Autodesk Inventor part; units mm, degrees
note: some values were not read from the file. Chosen so that the rebuilt part matches the saved one: direction of "Hole2".
(part 5 of 20)
  spline S27 degree 3 poles (-10071.861852, -10009.008209) (-10071.863963, -10009.012295) (-10071.868163, -10009.020425) (-10071.875194, -10009.032142) (-10071.882698, -10009.043397) (-10071.890711, -10009.054141) (-10071.899201, -10009.064358) (-10071.908156, -10009.074022) (-10071.917555, -10009.083111) (-10071.927381, -10009.091603) (-10071.937618, -10009.099474) (-10071.948247, -10009.1067) (-10071.95925, -10009.11326) (-10071.97061, -10009.119128) (-10071.982308, -10009.124286) (-10071.99433, -10009.128693) (-10072.006644, -10009.132397) (-10072.015041, -10009.134191) (-10072.019251, -10009.135091) knots 0 0 0 0 0.0658533 0.13104018 0.19559045 0.25953687 0.32291608 0.38576964 0.44814503 0.51009667 0.5716869 0.63298697 0.69407787 0.75505117 0.81600962 0.87706766 0.93835167 1 1 1 1
  spline S28 degree 3 poles (-10072.011557, -10009.107926) (-10072.008101, -10009.107314) (-10072.00122, -10009.106096) (-10071.991078, -10009.103593) (-10071.981148, -10009.100626) (-10071.971444, -10009.097167) (-10071.961973, -10009.093245) (-10071.949683, -10009.087429) (-10071.934919, -10009.079081) (-10071.91824, -10009.067495) (-10071.902707, -10009.054476) (-10071.888262, -10009.040263) (-10071.879682, -10009.029855) (-10071.875393, -10009.024653) knots 0 0 0 0 0.0644506 0.12832403 0.1917227 0.2547379 0.31744987 0.37992792 0.50437187 0.62845768 0.75238919 0.87624484 1 1 1 1
  spline S29 degree 3 poles (-10071.83509, -10008.810331) (-10071.836656, -10008.806851) (-10071.839768, -10008.799937) (-10071.84543, -10008.790125) (-10071.851743, -10008.780842) (-10071.858755, -10008.772119) (-10071.866422, -10008.763945) (-10071.874726, -10008.75632) (-10071.88364, -10008.749241) (-10071.89314, -10008.742705) (-10071.903202, -10008.736711) (-10071.913803, -10008.731254) (-10071.924919, -10008.726333) (-10071.936525, -10008.721945) (-10071.948599, -10008.718086) (-10071.961118, -10008.714764) (-10071.974052, -10008.711929) (-10071.982857, -10008.710502) (-10071.987308, -10008.70978) knots 0 0 0 0 0.05994656 0.11908522 0.17773662 0.23620436 0.29477068 0.35369309 0.41320222 0.47350071 0.53476324 0.59713734 0.66074485 0.72568383 0.79203056 0.85984183 0.92915698 1 1 1 1
  ellipse E534 centre (-10070.500516, -10008.838581) end of major axis (-10070.251393, -10008.817665) minor radius 0.13482 (-10070.407011, -10008.707729) -> (-10070.519101, -10008.704905) ccw
  ellipse E535 centre (-10070.496994, -10008.880539) end of major axis (-10070.746117, -10008.901455) minor radius 0.13482 (-10070.403489, -10008.749688) -> (-10070.515578, -10008.746863) ccw
  ellipse E536 centre (-10072.084336, -10008.798673) end of major axis (-10071.835212, -10008.777757) minor radius 0.13482 (-10071.990831, -10008.667822) -> (-10072.10292, -10008.664997) ccw
  ellipse E537 centre (-10072.080813, -10008.840632) end of major axis (-10072.329937, -10008.861548) minor radius 0.13482 (-10071.987308, -10008.70978) -> (-10072.099397, -10008.706956) ccw
  ellipse E538 centre (-10070.500714, -10008.942088) end of major axis (-10070.260175, -10009.010215) minor radius 0.20633 (-10070.539378, -10009.145021) -> (-10070.427738, -10009.147833) ccw
  ellipse E539 centre (-10072.084533, -10008.902181) end of major axis (-10071.843995, -10008.970307) minor radius 0.20633 (-10072.123197, -10009.105113) -> (-10072.011557, -10009.107926) ccw
  ellipse E540 centre (-10070.189892, -10008.99624) end of major axis (-10070.182637, -10008.708332) minor radius 0.048213 (-10070.237615, -10008.979123) -> (-10070.234208, -10009.15271) ccw
  ellipse E541 centre (-10070.189892, -10008.99624) end of major axis (-10070.182637, -10008.708332) minor radius 0.048213 (-10070.210183, -10008.754558) -> (-10070.231383, -10008.882208) ccw
  ellipse E542 centre (-10070.189892, -10008.99624) end of major axis (-10070.198405, -10009.334133) minor radius 0.056583 (-10070.213706, -10008.7126) -> (-10070.243358, -10008.923084) ccw
  ellipse E543 centre (-10070.189892, -10008.99624) end of major axis (-10070.198405, -10009.334133) minor radius 0.056583 (-10070.247084, -10009.05145) -> (-10070.241901, -10009.179875) ccw
  ellipse E544 centre (-10072.272412, -10008.943767) end of major axis (-10072.280926, -10009.28166) minor radius 0.056583 (-10072.296226, -10008.660127) -> (-10072.328408, -10008.92331) ccw
  ellipse E545 centre (-10072.272412, -10008.943767) end of major axis (-10072.280926, -10009.28166) minor radius 0.056583 (-10072.328363, -10009.061132) -> (-10072.324422, -10009.127402) ccw
  line L650 (-10070.153656, -10008.500579) -> (-10070.213706, -10008.7126)
  line L651 (-10072.296226, -10008.660127) -> (-10072.287518, -10008.62938)
  line L652 (-10072.262582, -10008.541339) -> (-10072.234911, -10008.443639)
  line L653 (-10070.156321, -10008.564386) -> (-10070.210183, -10008.754558)
  line L654 (-10070.55463, -10029.843391) -> (-10070.696895, -10029.517678)
  line L655 (-10070.813455, -10029.48076) -> (-10072.002453, -10029.540872)
  line L656 (-10072.082423, -10029.587726) -> (-10071.918753, -10029.962444)
  ellipse E546 centre (-10072.164414, -10029.974864) end of major axis (-10071.914557, -10029.983317) minor radius 0.10517 (-10072.058984, -10030.073195) -> (-10071.918753, -10029.962444) ccw
  line L657 (-10072.00092, -10029.495538) -> (-10070.811921, -10029.435426)
  line L658 (-10070.695362, -10029.472344) -> (-10070.552849, -10029.798623)
  line L659 (-10072.218164, -10030.077205) -> (-10072.218062, -10030.074202)
  ellipse E547 centre (-10070.79516, -10029.522646) end of major axis (-10070.695217, -10029.526028) minor radius 0.042068 (-10070.696895, -10029.517678) -> (-10070.813455, -10029.48076) ccw
  ellipse E548 centre (-10071.984158, -10029.582758) end of major axis (-10072.084101, -10029.579377) minor radius 0.042068 (-10072.002453, -10029.540872) -> (-10072.082423, -10029.587726) ccw
  ellipse E549 centre (-10070.793626, -10029.477312) end of major axis (-10070.693683, -10029.480693) minor radius 0.042068 (-10070.695362, -10029.472344) -> (-10070.811921, -10029.435426) ccw
  ellipse E550 centre (-10071.982624, -10029.537424) end of major axis (-10072.082567, -10029.534042) minor radius 0.042068 (-10072.00092, -10029.495538) -> (-10072.082567, -10029.534042) ccw
  line L660 (-10072.084101, -10029.579377) -> (-10072.082567, -10029.534042)
  ellipse E551 centre (-10071.975038, -10009.508335) end of major axis (-10072.07426, -10009.520779) minor radius 0.05049 (-10072.064562, -10009.494579) -> (-10072.074385, -10009.519539) ccw
  line L661 (-10072.074385, -10009.519539) -> (-10072.0701, -10009.575875)
  line L662 (-10070.209844, -10008.872593) -> (-10070.200885, -10009.028429)
  line L663 (-10070.19765, -10008.903676) -> (-10070.201202, -10008.841896)
  ellipse E552 centre (-10070.474229, -10008.585578) end of major axis (-10070.710151, -10008.502868) minor radius 0.210338 (-10070.421591, -10008.799368) -> (-10070.406555, -10008.797487) ccw
  ellipse E553 centre (-10070.474229, -10008.585578) end of major axis (-10070.710151, -10008.502868) minor radius 0.210338 (-10070.517863, -10008.79186) -> (-10070.489497, -10008.797511) ccw
  ellipse E554 centre (-10072.053337, -10008.505744) end of major axis (-10072.289259, -10008.423033) minor radius 0.210338 (-10072.096971, -10008.712025) -> (-10071.985663, -10008.717652) ccw
  spline S30 degree 3 poles (-10070.658378, -10008.462088) (-10070.660893, -10008.465426) (-10070.665904, -10008.472077) (-10070.672505, -10008.482647) (-10070.678344, -10008.493573) (-10070.683324, -10008.504882) (-10070.687423, -10008.516542) (-10070.6906, -10008.528536) (-10070.692819, -10008.540843) (-10070.694041, -10008.553443) (-10070.694229, -10008.566316) (-10070.693347, -10008.57944) (-10070.691363, -10008.592763) (-10070.688288, -10008.606105) (-10070.684175, -10008.619277) (-10070.679073, -10008.632108) (-10070.673107, -10008.6446) (-10070.668416, -10008.652554) (-10070.666066, -10008.65654) knots 0 0 0 0 0.06027236 0.12008459 0.17956335 0.23886314 0.2981675 0.35768957 0.41767151 0.47838294 0.54011829 0.60319317 0.66794006 0.7342313 0.80052522 0.86682566 0.93327954 1 1 1 1
  spline S31 degree 3 poles (-10070.553356, -10008.75156) (-10070.549759, -10008.753068) (-10070.542561, -10008.756086) (-10070.531515, -10008.760002) (-10070.520313, -10008.763504) (-10070.512721, -10008.765406) (-10070.508922, -10008.766357) knots 0 0 0 0 0.24945299 0.49932153 0.74952532 1 1 1 1
  spline S32 degree 3 poles (-10070.517863, -10008.79186) (-10070.520982, -10008.790973) (-10070.52722, -10008.789198) (-10070.536403, -10008.78595) (-10070.545444, -10008.782294) (-10070.554323, -10008.7782) (-10070.563034, -10008.773697) (-10070.571562, -10008.76879) (-10070.579921, -10008.763524) (-10070.585309, -10008.759719) (-10070.588009, -10008.757812) knots 0 0 0 0 0.12403661 0.24815991 0.37248981 0.49712476 0.62214288 0.74760322 0.87354721 1 1 1 1
  spline S33 degree 3 poles (-10070.659186, -10008.680563) (-10070.661891, -10008.676068) (-10070.667299, -10008.667078) (-10070.674475, -10008.653073) (-10070.680926, -10008.638751) (-10070.686555, -10008.624125) (-10070.691345, -10008.609262) (-10070.695259, -10008.594213) (-10070.698263, -10008.579033) (-10070.700325, -10008.563777) (-10070.701411, -10008.548499) (-10070.701486, -10008.533254) (-10070.700517, -10008.518096) (-10070.698468, -10008.503081) (-10070.695312, -10008.488261) (-10070.691008, -10008.473784) (-10070.685711, -10008.459784) (-10070.681307, -10008.45092) (-10070.679128, -10008.446533) knots 0 0 0 0 0.06405989 0.1281006 0.19204727 0.25582983 0.3193861 0.38266496 0.44562961 0.50826114 0.57056212 0.63256041 0.69431295 0.75590946 0.81747579 0.87917562 0.94021367 1 1 1 1
  spline S34 degree 3 poles (-10070.221275, -10008.458866) (-10070.219936, -10008.463284) (-10070.217233, -10008.4722) (-10070.214262, -10008.486006) (-10070.212053, -10008.500229) (-10070.210703, -10008.514871) (-10070.210204, -10008.529896) (-10070.210576, -10008.545278) (-10070.211832, -10008.56099) (-10070.213987, -10008.577004) (-10070.217057, -10008.593287) (-10070.221003, -10008.609667) (-10070.225831, -10008.625884) (-10070.231498, -10008.641687) (-10070.237946, -10008.656979) (-10070.245168, -10008.671706) (-10070.253061, -10008.685881) (-10070.258963, -10008.694864) (-10070.261897, -10008.699331) knots 0 0 0 0 0.0549764 0.11096338 0.16806833 0.22639244 0.28603139 0.34707614 0.40961367 0.47372767 0.53949927 0.6069434 0.67436537 0.7409998 0.80686402 0.87197412 0.93634658 1 1 1 1
  spline S35 degree 3 poles (-10070.331636, -10008.768087) (-10070.334512, -10008.769872) (-10070.340254, -10008.773436) (-10070.349165, -10008.778254) (-10070.358264, -10008.782658) (-10070.367565, -10008.786598) (-10070.377053, -10008.790076) (-10070.386722, -10008.793065) (-10070.396556, -10008.795599) (-10070.403217, -10008.796857) (-10070.406555, -10008.797487) knots 0 0 0 0 0.12529925 0.25024005 0.37494166 0.49953681 0.62417216 0.7490086 0.87422136 1 1 1 1
  spline S36 degree 3 poles (-10070.397614, -10008.771984) (-10070.395674, -10008.771696) (-10070.391803, -10008.771121) (-10070.386046, -10008.77004) (-10070.380348, -10008.768808) (-10070.374712, -10008.767411) (-10070.36914, -10008.765857) (-10070.363634, -10008.764146) (-10070.35819, -10008.762293) (-10070.354613, -10008.760932) (-10070.352826, -10008.760251) knots 0 0 0 0 0.12682999 0.25300914 0.37860655 0.50368723 0.62831214 0.75253809 0.87641783 1 1 1 1
  spline S37 degree 3 poles (-10070.212712, -10008.477821) (-10070.213431, -10008.476078) (-10070.214864, -10008.472607) (-10070.217274, -10008.467539) (-10070.219844, -10008.462594) (-10070.221723, -10008.459403) (-10070.22266, -10008.457812) knots 0 0 0 0 0.25282857 0.50351543 0.75244628 1 1 1 1
  spline S38 degree 3 poles (-10072.269159, -10008.447042) (-10072.26983, -10008.450164) (-10072.271179, -10008.456431) (-10072.272459, -10008.466017) (-10072.273184, -10008.475761) (-10072.273284, -10008.485667) (-10072.272755, -10008.495721) (-10072.271577, -10008.505916) (-10072.269742, -10008.516207) (-10072.267263, -10008.526488) (-10072.264171, -10008.536647) (-10072.260499, -10008.546609) (-10072.256269, -10008.556358) (-10072.251502, -10008.565881) (-10072.246221, -10008.575168) (-10072.240438, -10008.584198) (-10072.234209, -10008.592987) (-10072.229695, -10008.598589) (-10072.227432, -10008.601397) knots 0 0 0 0 0.05778221 0.11602992 0.17490487 0.23457915 0.29523385 0.35705764 0.42024514 0.48436692 0.54838884 0.61238964 0.67645987 0.74067474 0.80509501 0.86976792 0.93472837 1 1 1 1
  spline S39 degree 3 poles (-10072.096971, -10008.712025) (-10072.098084, -10008.71172) (-10072.100309, -10008.711109) (-10072.103625, -10008.710118) (-10072.106926, -10008.709075) (-10072.109111, -10008.708331) (-10072.110204, -10008.707959) knots 0 0 0 0 0.24996578 0.49993063 0.74993068 1 1 1 1
  spline S40 degree 3 poles (-10072.220944, -10008.625594) (-10072.22586, -10008.618945) (-10072.235704, -10008.605633) (-10072.248247, -10008.584162) (-10072.259045, -10008.561811) (-10072.267812, -10008.538671) (-10072.274461, -10008.514988) (-10072.278121, -10008.494921) (-10072.279848, -10008.478814) (-10072.280512, -10008.466755) (-10072.280592, -10008.454718) (-10072.280093, -10008.446728) (-10072.279843, -10008.442739) knots 0 0 0 0 0.12626187 0.25278671 0.37919835 0.50514032 0.63031299 0.75451273 0.81623998 0.87771389 0.93895544 1 1 1 1
  spline S41 degree 3 poles (-10071.789522, -10008.445235) (-10071.789556, -10008.453662) (-10071.789607, -10008.466432) (-10071.791265, -10008.483554) (-10071.793068, -10008.496725) (-10071.795505, -10008.510082) (-10071.799565, -10008.528079) (-10071.806062, -10008.550228) (-10071.816137, -10008.575732) (-10071.828254, -10008.599763) (-10071.840038, -10008.61848) (-10071.850323, -10008.63256) (-10071.855843, -10008.639206) (-10071.858591, -10008.642514) knots 0 0 0 0 0.11836757 0.17935651 0.24161124 0.30518476 0.370129 0.50087366 0.62916185 0.75504201 0.87860366 0.93956774 1 1 1 1
  spline S42 degree 3 poles (-10071.9666, -10008.713362) (-10071.968168, -10008.713786) (-10071.971306, -10008.714634) (-10071.976057, -10008.715757) (-10071.980841, -10008.716781) (-10071.984054, -10008.717362) (-10071.985663, -10008.717652) knots 0 0 0 0 0.24922132 0.49890182 0.74913063 1 1 1 1
  ellipse E555 centre (-10070.465288, -10008.560076) end of major axis (-10070.229367, -10008.642786) minor radius 0.210338 (-10070.508922, -10008.766357) -> (-10070.473977, -10008.772907) ccw
  ellipse E556 centre (-10070.465288, -10008.560076) end of major axis (-10070.229367, -10008.642786) minor radius 0.210338 (-10070.419103, -10008.774408) -> (-10070.397614, -10008.771984) ccw
  ellipse E557 centre (-10070.153161, -10008.634844) end of major axis (-10070.138619, -10008.347212) minor radius 0.051474 (-10070.206261, -10008.740713) -> (-10070.204743, -10008.780269) ccw
  ellipse E558 centre (-10070.153161, -10008.634844) end of major axis (-10070.138619, -10008.347212) minor radius 0.051474 (-10070.185488, -10008.459786) -> (-10070.206118, -10008.673328) ccw
  ellipse E559 centre (-10070.153161, -10008.634844) end of major axis (-10070.170227, -10008.972413) minor radius 0.06041 (-10070.195395, -10008.454067) -> (-10070.215733, -10008.702837) ccw
  ellipse E560 centre (-10070.153161, -10008.634844) end of major axis (-10070.170227, -10008.972413) minor radius 0.06041 (-10070.215082, -10008.77388) -> (-10070.213724, -10008.80505) ccw
  ellipse E561 centre (-10072.229486, -10008.529872) end of major axis (-10072.246552, -10008.867441) minor radius 0.06041 (-10072.283768, -10008.443881) -> (-10072.291977, -10008.645125) ccw
  line L664 (-10070.21001, -10007.456492) -> (-10070.103322, -10007.152174)
  line L665 (-10070.183704, -10007.096201) -> (-10071.372703, -10007.036089)
  line L666 (-10071.488849, -10007.082126) -> (-10071.595537, -10007.386444)
  line L667 (-10070.100854, -10007.19511) -> (-10070.192795, -10007.457362)
  ellipse E562 centre (-10070.201586, -10007.147206) end of major axis (-10070.101751, -10007.141467) minor radius 0.051008 (-10070.103322, -10007.152174) -> (-10070.183704, -10007.096201) ccw
  ellipse E563 centre (-10071.390585, -10007.087094) end of major axis (-10071.49042, -10007.092833) minor radius 0.051008 (-10071.372703, -10007.036089) -> (-10071.488849, -10007.082126) ccw
  ellipse E564 centre (-10070.199118, -10007.190142) end of major axis (-10070.099283, -10007.184403) minor radius 0.051008 (-10070.100854, -10007.19511) -> (-10070.099283, -10007.184403) ccw
  line L668 (-10070.101751, -10007.141467) -> (-10070.099283, -10007.184403)
  line L669 (-10070.217767, -10029.383474) -> (-10070.202807, -10029.429786)
  line L670 (-10072.250735, -10029.563465) -> (-10072.304434, -10029.397224)
  line L671 (-10070.214557, -10029.338695) -> (-10070.200574, -10029.381982)
  line L672 (-10070.217767, -10029.383474) -> (-10070.318002, -10029.384134)
  ellipse E565 centre (-10070.353925, -10029.272923) end of major axis (-10070.603286, -10029.255048) minor radius 0.110059 (-10070.60081, -10029.27455) -> (-10070.318002, -10029.384134) ccw
  line L673 (-10070.60081, -10029.27455) -> (-10070.72936, -10028.876586)
  line L674 (-10070.842483, -10028.832753) -> (-10072.037404, -10028.840627)
  line L675 (-10072.121788, -10028.885762) -> (-10072.024288, -10029.187602)
  ellipse E566 centre (-10072.240122, -10029.285352) end of major axis (-10072.489483, -10029.267477) minor radius 0.110059 (-10072.204199, -10029.396563) -> (-10072.064381, -10029.373778) ccw
  line L676 (-10072.204199, -10029.396563) -> (-10072.304434, -10029.397224)
  line L677 (-10072.034194, -10028.795847) -> (-10070.839273, -10028.787973)
  line L678 (-10072.301224, -10029.352445) -> (-10072.200989, -10029.351784)
  ellipse E567 centre (-10072.236912, -10029.240573) end of major axis (-10071.987552, -10029.258448) minor radius 0.110059 (-10072.200989, -10029.351784) -> (-10072.080406, -10029.335495) ccw
  line L679 (-10070.72615, -10028.831807) -> (-10070.5976, -10029.229771)
  ellipse E568 centre (-10070.350715, -10029.228144) end of major axis (-10070.600076, -10029.210269) minor radius 0.110059 (-10070.5976, -10029.229771) -> (-10070.314792, -10029.339355) ccw
  line L680 (-10070.314792, -10029.339355) -> (-10070.214557, -10029.338695)
  line L681 (-10072.304434, -10029.397224) -> (-10072.301224, -10029.352445)
  line L682 (-10070.214557, -10029.338695) -> (-10070.217767, -10029.383474)
  ellipse E569 centre (-10070.828114, -10028.877237) end of major axis (-10070.72837, -10028.884387) minor radius 0.044024 (-10070.72936, -10028.876586) -> (-10070.842483, -10028.832753) ccw
  ellipse E570 centre (-10072.023034, -10028.885111) end of major axis (-10072.122778, -10028.877961) minor radius 0.044024 (-10072.037404, -10028.840627) -> (-10072.121788, -10028.885762) ccw
  ellipse E571 centre (-10070.824904, -10028.832458) end of major axis (-10070.72516, -10028.839608) minor radius 0.044024 (-10070.72615, -10028.831807) -> (-10070.839273, -10028.787973) ccw
  ellipse E572 centre (-10072.019824, -10028.840332) end of major axis (-10072.119568, -10028.833182) minor radius 0.044024 (-10072.034194, -10028.795847) -> (-10072.119568, -10028.833182) ccw
  line L683 (-10072.122778, -10028.877961) -> (-10072.119568, -10028.833182)
  line L684 (-10070.255655, -10009.359471) -> (-10070.253325, -10009.387391)
  line L685 (-10072.342322, -10009.345721) -> (-10072.324967, -10009.553657)
  line L686 (-10070.244545, -10009.38407) -> (-10070.24867, -10009.334658)
  ellipse E573 centre (-10070.523146, -10009.14643) end of major axis (-10070.763791, -10009.078681) minor radius 0.214215 (-10070.561433, -10009.357456) -> (-10070.449571, -10009.358193) ccw
  ellipse E574 centre (-10072.110119, -10009.135972) end of major axis (-10072.350764, -10009.068224) minor radius 0.214215 (-10072.148406, -10009.346999) -> (-10072.036544, -10009.347736) ccw
  spline S43 degree 3 poles (-10070.535305, -10008.939692) (-10070.548916, -10008.941587) (-10070.575744, -10008.945323) (-10070.613933, -10008.957678) (-10070.648934, -10008.974395) (-10070.679956, -10008.995533) (-10070.706251, -10009.02058) (-10070.727025, -10009.049184) (-10070.739022, -10009.075696) (-10070.744924, -10009.097975) (-10070.747464, -10009.115295) (-10070.748005, -10009.133142) (-10070.74645, -10009.151455) (-10070.742731, -10009.170025) (-10070.73692, -10009.188455) (-10070.72914, -10009.206337) (-10070.716362, -10009.229167) (-10070.696166, -10009.25554) (-10070.666542, -10009.282862) (-10070.632398, -10009.305299) (-10070.594835, -10009.322849) (-10070.567944, -10009.32937) (-10070.554448, -10009.332643) knots 0 0 0 0 0.06705351 0.13217076 0.19521445 0.25608707 0.314845 0.37183317 0.42783149 0.45589727 0.48426542 0.51319288 0.54296576 0.57389196 0.60556318 0.63723227 0.66902668 0.73324746 0.79861392 0.865047 0.93227307 1 1 1 1
  spline S44 degree 3 poles (-10070.561433, -10009.357456) (-10070.568232, -10009.355693) (-10070.581851, -10009.352162) (-10070.6081, -10009.341466) (-10070.639159, -10009.323392) (-10070.672368, -10009.295199) (-10070.701073, -10009.261778) (-10070.72456, -10009.224269) (-10070.74211, -10009.183833) (-10070.752969, -10009.141615) (-10070.755774, -10009.105721) (-10070.753806, -10009.077427) (-10070.750159, -10009.056625) (-10070.744322, -10009.036588) (-10070.736454, -10009.017672) (-10070.726747, -10009.00014) (-10070.711608, -10008.978693) (-10070.688601, -10008.955108) (-10070.655962, -10008.932353) (-10070.619434, -10008.915032) (-10070.580116, -10008.902519) (-10070.55273, -10008.898374) (-10070.538928, -10008.896284) knots 0 0 0 0 0.03133748 0.06278121 0.12629735 0.19093644 0.25645898 0.32231967 0.3878749 0.45257734 0.51618281 0.54767829 0.57907039 0.61032535 0.64070557 0.67038635 0.69964994 0.75776174 0.81647804 0.87644136 0.93772561 1 1 1 1
  spline S45 degree 3 poles (-10070.426615, -10008.897024) (-10070.414157, -10008.899384) (-10070.389891, -10008.903981) (-10070.356516, -10008.918864) (-10070.32752, -10008.93892) (-10070.303357, -10008.964177) (-10070.284368, -10008.993979) (-10070.270883, -10009.027844) (-10070.263206, -10009.065261) (-10070.261642, -10009.105753) (-10070.26644, -10009.148364) (-10070.277295, -10009.19114) (-10070.294334, -10009.231769) (-10070.316718, -10009.268453) (-10070.343921, -10009.300386) (-10070.370323, -10009.322476) (-10070.393242, -10009.336867) (-10070.411248, -10009.345895) (-10070.430019, -10009.353272) (-10070.443044, -10009.35655) (-10070.449571, -10009.358193) knots 0 0 0 0 0.06022667 0.11730293 0.17254203 0.22724068 0.28263107 0.33984452 0.39989686 0.46369518 0.53205848 0.6034638 0.67318901 0.7411164 0.8073508 0.87214279 0.90417982 0.93607992 0.96796844 1 1 1 1
  spline S46 degree 3 poles (-10070.442585, -10009.33338) (-10070.439287, -10009.332715) (-10070.432714, -10009.33139) (-10070.423031, -10009.328782) (-10070.413541, -10009.325749) (-10070.401189, -10009.321112) (-10070.386253, -10009.314249) (-10070.369219, -10009.304429) (-10070.353144, -10009.293184) (-10070.33811, -10009.280626) (-10070.324062, -10009.266975) (-10070.315642, -10009.257018) (-10070.311433, -10009.252041) knots 0 0 0 0 0.06406043 0.12763921 0.19082759 0.25370622 0.37876994 0.50330734 0.62760512 0.75181377 0.87596664 1 1 1 1
  spline S47 degree 3 poles (-10070.265966, -10009.03859) (-10070.267502, -10009.035036) (-10070.270547, -10009.027987) (-10070.276209, -10009.018024) (-10070.282579, -10009.008657) (-10070.28971, -10008.999913) (-10070.297553, -10008.991776) (-10070.306084, -10008.984241) (-10070.315273, -10008.977301) (-10070.325093, -10008.970948) (-10070.335516, -10008.965174) (-10070.346515, -10008.959971) (-10070.358062, -10008.955331) (-10070.370131, -10008.951249) (-10070.382695, -10008.947712) (-10070.395728, -10008.944726) (-10070.409198, -10008.942236) (-10070.418358, -10008.941038) (-10070.422992, -10008.940432) knots 0 0 0 0 0.05963345 0.11825449 0.17626219 0.23403402 0.29191894 0.35023204 0.40925111 0.46921525 0.53032509 0.59274441 0.65660269 0.7219981 0.78900076 0.85765603 0.92798753 1 1 1 1
  spline S48 degree 3 poles (-10072.122278, -10008.929235) (-10072.135889, -10008.93113) (-10072.162717, -10008.934866) (-10072.200906, -10008.947221) (-10072.235907, -10008.963938) (-10072.266929, -10008.985076) (-10072.293224, -10009.010123) (-10072.313998, -10009.038727) (-10072.325995, -10009.065239) (-10072.331897, -10009.087518) (-10072.334437, -10009.104838) (-10072.334978, -10009.122685) (-10072.333423, -10009.140998) (-10072.329704, -10009.159568) (-10072.323893, -10009.177998) (-10072.316113, -10009.19588) (-10072.303335, -10009.21871) (-10072.283139, -10009.245083) (-10072.253515, -10009.272405) (-10072.219371, -10009.294841) (-10072.181808, -10009.312391) (-10072.154917, -10009.318913) (-10072.141421, -10009.322186) knots 0 0 0 0 0.06705351 0.13217076 0.19521445 0.25608707 0.314845 0.37183317 0.42783149 0.45589727 0.48426542 0.51319288 0.54296576 0.57389196 0.60556318 0.63723227 0.66902668 0.73324746 0.79861392 0.865047 0.93227307 1 1 1 1
  spline S49 degree 3 poles (-10072.148406, -10009.346999) (-10072.155205, -10009.345236) (-10072.168824, -10009.341705) (-10072.195073, -10009.331009) (-10072.226132, -10009.312934) (-10072.259341, -10009.284741) (-10072.288046, -10009.251321) (-10072.311533, -10009.213812) (-10072.329083, -10009.173376) (-10072.339942, -10009.131158) (-10072.342747, -10009.095264) (-10072.340779, -10009.06697) (-10072.337132, -10009.046168) (-10072.331295, -10009.02613) (-10072.323427, -10009.007215) (-10072.31372, -10008.989683) (-10072.298581, -10008.968236) (-10072.275574, -10008.944651) (-10072.242935, -10008.921896) (-10072.206408, -10008.904574) (-10072.167089, -10008.892062) (-10072.139703, -10008.887916) (-10072.125901, -10008.885827) knots 0 0 0 0 0.03133748 0.06278121 0.12629735 0.19093644 0.25645898 0.32231967 0.3878749 0.45257734 0.51618281 0.54767829 0.57907039 0.61032535 0.64070557 0.67038635 0.69964994 0.75776174 0.81647804 0.87644136 0.93772561 1 1 1 1
  spline S50 degree 3 poles (-10072.013588, -10008.886567) (-10072.00113, -10008.888927) (-10071.976864, -10008.893523) (-10071.943489, -10008.908407) (-10071.914493, -10008.928463) (-10071.890331, -10008.953719) (-10071.871341, -10008.983521) (-10071.857856, -10009.017387) (-10071.850179, -10009.054804) (-10071.848616, -10009.095296) (-10071.853413, -10009.137907) (-10071.864268, -10009.180683) (-10071.881307, -10009.221312) (-10071.903691, -10009.257996) (-10071.930894, -10009.289929) (-10071.957296, -10009.312019) (-10071.980216, -10009.32641) (-10071.998221, -10009.335438) (-10072.016992, -10009.342815) (-10072.030017, -10009.346093) (-10072.036544, -10009.347736) knots 0 0 0 0 0.06022667 0.11730293 0.17254203 0.22724068 0.28263107 0.33984452 0.39989686 0.46369518 0.53205848 0.6034638 0.67318901 0.7411164 0.8073508 0.87214279 0.90417982 0.93607992 0.96796844 1 1 1 1
  spline S51 degree 3 poles (-10072.029558, -10009.322923) (-10072.02626, -10009.322258) (-10072.019687, -10009.320933) (-10072.010004, -10009.318325) (-10072.000514, -10009.315292) (-10071.988162, -10009.310655) (-10071.973226, -10009.303792) (-10071.956192, -10009.293972) (-10071.940117, -10009.282726) (-10071.925083, -10009.270168) (-10071.911035, -10009.256518) (-10071.902615, -10009.24656) (-10071.898406, -10009.241584) knots 0 0 0 0 0.06406043 0.12763921 0.19082759 0.25370622 0.37876994 0.50330734 0.62760512 0.75181377 0.87596664 1 1 1 1
  spline S52 degree 3 poles (-10071.852939, -10009.028133) (-10071.854475, -10009.024578) (-10071.85752, -10009.01753) (-10071.863182, -10009.007567) (-10071.869552, -10008.9982) (-10071.876683, -10008.989456) (-10071.884526, -10008.981319) (-10071.893057, -10008.973784) (-10071.902246, -10008.966844) (-10071.912066, -10008.960491) (-10071.922489, -10008.954717) (-10071.933488, -10008.949514) (-10071.945035, -10008.944874) (-10071.957104, -10008.940791) (-10071.969668, -10008.937254) (-10071.982701, -10008.934268) (-10071.996171, -10008.931778) (-10072.005331, -10008.930581) (-10072.009965, -10008.929975) knots 0 0 0 0 0.05963345 0.11825449 0.17626219 0.23403402 0.29191894 0.35023204 0.40925111 0.46921525 0.53032509 0.59274441 0.65660269 0.7219981 0.78900076 0.85765603 0.92798753 1 1 1 1
  ellipse E575 centre (-10070.516783, -10009.017467) end of major axis (-10070.26765, -10008.996673) minor radius 0.122746 (-10070.426615, -10008.897024) -> (-10070.538928, -10008.896284) ccw
  ellipse E576 centre (-10070.513161, -10009.060874) end of major axis (-10070.762294, -10009.081668) minor radius 0.122746 (-10070.422992, -10008.940432) -> (-10070.535305, -10008.939692) ccw
  ellipse E577 centre (-10072.103757, -10009.007009) end of major axis (-10071.854623, -10008.986216) minor radius 0.122746 (-10072.013588, -10008.886567) -> (-10072.125901, -10008.885827) ccw
  ellipse E578 centre (-10072.100134, -10009.050417) end of major axis (-10072.349267, -10009.071211) minor radius 0.122746 (-10072.009965, -10008.929975) -> (-10072.122278, -10008.929235) ccw
  ellipse E579 centre (-10070.516161, -10009.121617) end of major axis (-10070.275515, -10009.189365) minor radius 0.214215 (-10070.554448, -10009.332643) -> (-10070.442585, -10009.33338) ccw
  ellipse E580 centre (-10072.103134, -10009.11116) end of major axis (-10071.862488, -10009.178908) minor radius 0.214215 (-10072.141421, -10009.322186) -> (-10072.029558, -10009.322923) ccw
  ellipse E581 centre (-10070.208433, -10009.191736) end of major axis (-10070.206535, -10008.903742) minor radius 0.045287 (-10070.229301, -10008.941708) -> (-10070.24867, -10009.334658) ccw
  ellipse E582 centre (-10070.208433, -10009.191736) end of major axis (-10070.21066, -10009.529728) minor radius 0.05315 (-10070.232924, -10008.898301) -> (-10070.255655, -10009.359471) ccw
  ellipse E583 centre (-10072.2951, -10009.177986) end of major axis (-10072.297327, -10009.515978) minor radius 0.05315 (-10072.319592, -10008.884551) -> (-10072.342322, -10009.345721) ccw
  line L687 (-10070.188103, -10008.739092) -> (-10070.232924, -10008.898301)
  line L688 (-10072.319592, -10008.884551) -> (-10072.314908, -10008.867915)
  line L689 (-10072.310488, -10008.852215) -> (-10072.306859, -10008.839323)
  line L690 (-10070.184093, -10008.781125) -> (-10070.229301, -10008.941708)
  line L691 (-10072.287124, -10029.657627) -> (-10072.28215, -10029.55113)
  ellipse E584 centre (-10072.614332, -10008.63776) end of major axis (-10072.316064, -10008.722237) minor radius 0.255849 (-10072.308804, -10008.645459) -> (-10072.310399, -10008.631601) ccw
  line L692 (-10072.310399, -10008.631601) -> (-10072.291341, -10008.56431)
  line L693 (-10072.304638, -10008.695072) -> (-10072.308804, -10008.645459)
  arc A6 (-10072.145042, -10030.918218) -> (-10072.035081, -10030.817063) centre (-10072.293754, -10030.646216) ccw
  ellipse E585 centre (-10072.198448, -10008.642704) end of major axis (-10072.176105, -10008.200769) minor radius 0.079087 (-10072.259382, -10008.443478) -> (-10072.261023, -10008.455542) ccw
  arc A7 (-10072.040297, -10007.363958) -> (-10072.162646, -10007.238636) centre (-10072.314255, -10007.509034) ccw
  ellipse E586 centre (-10072.634569, -10029.367064) end of major axis (-10072.339577, -10029.271776) minor radius 0.274042 (-10072.329925, -10029.379827) -> (-10072.328432, -10029.365047) ccw
  line L694 (-10072.324956, -10029.395211) -> (-10072.329925, -10029.379827)
  line L695 (-10072.328432, -10029.365047) -> (-10072.318432, -10029.22554)
  ellipse E587 centre (-10072.667728, -10009.440187) end of major axis (-10072.358802, -10009.414403) minor radius 0.152204 (-10072.364524, -10009.450886) -> (-10072.361591, -10009.442204) ccw
  line L696 (-10072.356199, -10009.550633) -> (-10072.364524, -10009.450886)
  ellipse E588 centre (-10072.640059, -10008.876501) end of major axis (-10072.341659, -10008.960508) minor radius 0.265627 (-10072.333923, -10008.878518) -> (-10072.335552, -10008.86419) ccw
  line L697 (-10072.335552, -10008.86419) -> (-10072.32153, -10008.814384)
  line L698 (-10072.329624, -10008.930018) -> (-10072.333923, -10008.878518)
  line L699 (-10072.361591, -10009.442204) -> (-10072.34674, -10009.389452)
  ellipse E589 centre (-10072.268637, -10009.299414) end of major axis (-10072.265721, -10008.856923) minor radius 0.069582 (-10072.327582, -10009.079251) -> (-10072.329926, -10009.105362) ccw
  arc A8 (-10070.204089, -10029.45722) -> (-10070.180383, -10029.591386) centre (-10069.894426, -10029.471684) ccw
  line L700 (-10070.180383, -10029.591386) -> (-10070.161234, -10029.637131)
  line L701 (-10070.188871, -10029.131404) -> (-10070.204089, -10029.45722)
  arc A9 (-10070.153135, -10029.863748) -> (-10070.146971, -10029.878943) centre (-10069.862888, -10029.754861) ccw
  arc A10 (-10070.17271, -10029.744379) -> (-10070.162129, -10029.835822) centre (-10069.862888, -10029.754861) ccw
  line L702 (-10070.146971, -10029.878943) -> (-10070.107583, -10029.969123)
  line L703 (-10070.168495, -10029.619785) -> (-10070.17271, -10029.744379)
  arc A11 (-10064.803665, -10028.498381) -> (-10064.804405, -10028.496309) centre (-10065.93415, -10028.900878) ccw
  line L704 (-10065.739572, -10009.914301) -> (-10064.795739, -10009.815465)
  line L705 (-10065.739572, -10028.279681) -> (-10064.795739, -10028.378516)
  arc A12 (-10064.804405, -10009.697673) -> (-10064.803665, -10009.695601) centre (-10065.93415, -10009.293103) ccw
  arc A13 (-10061.963392, -10012.693942) -> (-10061.988959, -10012.57834) centre (-10063.146433, -10012.894969) ccw
  line L706 (-10063.254748, -10012.391479) -> (-10063.19647, -10012.37859)
  arc A14 (-10061.988959, -10025.615641) -> (-10061.963392, -10025.50004) centre (-10063.146433, -10025.299013) ccw
  line L707 (-10063.254748, -10025.802502) -> (-10063.19647, -10025.815392)
  arc A15 (-10062.980311, -10029.363176) -> (-10062.946041, -10028.8732) centre (-10064.134914, -10029.036234) ccw
  line L708 (-10075.604898, -10030.131778) -> (-10075.41751, -10030.122304)
  line L709 (-10074.395345, -10030.070627) -> (-10074.252598, -10030.06341)
  line L710 (-10068.108391, -10029.752778) -> (-10065.7939, -10029.635765)
  line L711 (-10064.717976, -10029.581369) -> (-10064.036436, -10029.546913)
  arc A16 (-10062.078316, -10026.449206) -> (-10062.072096, -10026.330858) centre (-10063.27209, -10026.327128) ccw
  line L712 (-10063.257788, -10025.812169) -> (-10063.19647, -10025.815392)
  line L713 (-10064.058103, -10026.801529) -> (-10063.101628, -10026.851798)
  line L714 (-10064.204708, -10013.589145) -> (-10064.127903, -10013.572866)
  arc A17 (-10061.758802, -10010.204911) -> (-10061.792515, -10009.905981) centre (-10062.958695, -10010.188867) ccw
  line L715 (-10063.773106, -10009.76245) -> (-10062.832424, -10009.656361)
  line L716 (-10063.665823, -10010.78688) -> (-10062.716995, -10010.679873)
  arc A18 (-10061.792515, -10028.288001) -> (-10061.758802, -10027.989071) centre (-10062.958695, -10028.005115) ccw
  line L717 (-10063.665823, -10027.407102) -> (-10062.716995, -10027.514109)
  line L718 (-10063.773106, -10028.431532) -> (-10062.832424, -10028.53762)
  line L719 (-10064.204708, -10024.604837) -> (-10064.127903, -10024.621116)
  arc A19 (-10062.072096, -10011.863124) -> (-10062.078316, -10011.744776) centre (-10063.27209, -10011.866854) ccw
  line L720 (-10064.058103, -10011.392453) -> (-10063.101628, -10011.342184)
  line L721 (-10063.257788, -10012.381813) -> (-10063.19647, -10012.37859)
  arc A20 (-10062.946041, -10009.320782) -> (-10062.980311, -10008.830805) centre (-10064.134914, -10009.157748) ccw
  line L722 (-10075.604898, -10008.062204) -> (-10075.41751, -10008.071677)
  line L723 (-10074.395345, -10008.123355) -> (-10074.285045, -10008.128931)
  line L724 (-10068.139186, -10008.439647) -> (-10065.7939, -10008.558217)
  line L725 (-10064.717976, -10008.612612) -> (-10064.036436, -10008.647069)
  line L726 (-10075.547709, -10028.283156) -> (-10075.506599, -10028.282885)
  line L727 (-10068.188087, -10028.234661) -> (-10067.69897, -10028.231438)
  line L728 (-10068.306944, -10010.104133) -> (-10066.77146, -10009.954131)
  line L729 (-10068.306944, -10028.089848) -> (-10066.77146, -10028.239851)
  line L730 (-10075.547709, -10009.910825) -> (-10075.506599, -10009.911096)
  line L731 (-10068.198721, -10009.959251) -> (-10067.69897, -10009.962544)
  ellipse E590 centre (-10081.309124, -10029.28828) end of major axis (-10081.266302, -10030.987741) minor radius 0.28459 (-10081.483986, -10030.474215) -> (-10081.266302, -10030.987741) ccw
  line L732 (-10081.112634, -10030.983869) -> (-10081.266302, -10030.987741)
  ellipse E591 centre (-10081.309124, -10008.905701) end of major axis (-10081.266302, -10007.206241) minor radius 0.28459 (-10081.266302, -10007.206241) -> (-10081.483986, -10007.719767) ccw
  line L733 (-10081.112634, -10007.210113) -> (-10081.266302, -10007.206241)
  ellipse E592 centre (-10079.464151, -10029.811232) end of major axis (-10079.378314, -10031.509063) minor radius 0.303839 (-10079.670137, -10030.759238) -> (-10079.378314, -10031.509063) ccw
  line L734 (-10079.234984, -10031.501817) -> (-10079.378314, -10031.509063)
  ellipse E593 centre (-10079.464151, -10008.38275) end of major axis (-10079.378314, -10006.684918) minor radius 0.303839 (-10079.378314, -10006.684918) -> (-10079.670137, -10007.434743) ccw
  line L735 (-10079.234984, -10006.692165) -> (-10079.378314, -10006.684918)
  ellipse E594 centre (-10082.380777, -10011.996464) end of major axis (-10082.546064, -10010.304519) minor radius 0.097712 (-10082.546064, -10010.304519) -> (-10082.565803, -10010.821909) ccw
  line L736 (-10082.296519, -10010.280141) -> (-10082.546064, -10010.304519)
  ellipse E595 centre (-10082.380777, -10026.197517) end of major axis (-10082.546064, -10027.889463) minor radius 0.097712 (-10082.565803, -10027.372073) -> (-10082.546064, -10027.889463) ccw
  line L737 (-10082.296519, -10027.913841) -> (-10082.546064, -10027.889463)
  ellipse E596 centre (-10078.25384, -10029.211297) end of major axis (-10078.291624, -10027.711772) minor radius 0.251109 (-10078.479438, -10028.338173) -> (-10078.507636, -10028.961756) ccw
  ellipse E597 centre (-10078.25384, -10029.211297) end of major axis (-10078.301699, -10027.311899) minor radius 0.318071 (-10078.557274, -10028.330023) -> (-10078.491317, -10030.275512) ccw
  ellipse E598 centre (-10081.013451, -10029.28083) end of major axis (-10080.965592, -10031.180227) minor radius 0.318071 (-10081.291909, -10029.982743) -> (-10080.965592, -10031.180227) ccw
  line L738 (-10079.586995, -10031.145491) -> (-10080.965592, -10031.180227)
  ellipse E599 centre (-10077.331965, -10011.646037) end of major axis (-10077.529845, -10009.75637) minor radius 0.08119 (-10077.480252, -10009.914538) -> (-10077.544789, -10009.973052) ccw
  ellipse E600 centre (-10080.114195, -10011.937384) end of major axis (-10080.312075, -10010.047717) minor radius 0.08119 (-10080.327672, -10010.158439) -> (-10080.314114, -10010.558943) ccw
  line L739 (-10077.529845, -10009.75637) -> (-10079.489123, -10009.96154)
  ellipse E601 centre (-10077.331965, -10026.547944) end of major axis (-10077.529845, -10028.437612) minor radius 0.08119 (-10077.544789, -10028.22093) -> (-10077.480252, -10028.279443) ccw
  ellipse E602 centre (-10080.114195, -10026.256598) end of major axis (-10080.312075, -10028.146265) minor radius 0.08119 (-10080.314114, -10027.635038) -> (-10080.327672, -10028.035542) ccw
  line L740 (-10077.529845, -10028.437612) -> (-10079.489123, -10028.232442)
  ellipse E603 centre (-10078.25384, -10008.982685) end of major axis (-10078.216057, -10007.483161) minor radius 0.251109 (-10078.507636, -10009.232226) -> (-10078.479438, -10009.855808) ccw
  ellipse E604 centre (-10078.25384, -10008.982685) end of major axis (-10078.205981, -10007.083288) minor radius 0.318071 (-10078.491317, -10007.91847) -> (-10078.557274, -10009.863959) ccw
  ellipse E605 centre (-10081.013451, -10008.913151) end of major axis (-10080.965592, -10007.013754) minor radius 0.318071 (-10080.965592, -10007.013754) -> (-10081.291909, -10008.211239) ccw
  line L741 (-10079.586995, -10007.048491) -> (-10080.965592, -10007.013754)
  ellipse E606 centre (-10076.417956, -10029.657226) end of major axis (-10076.342218, -10031.155313) minor radius 0.268093 (-10076.619894, -10028.376473) -> (-10076.196715, -10030.847573) ccw
  ellipse E607 centre (-10076.417956, -10029.657226) end of major axis (-10076.322021, -10031.554802) minor radius 0.339584 (-10076.730075, -10028.364047) -> (-10076.094418, -10030.842401) ccw
  ellipse E608 centre (-10079.169358, -10029.796328) end of major axis (-10079.073422, -10031.693905) minor radius 0.339584 (-10079.471363, -10030.311689) -> (-10079.073422, -10031.693905) ccw
  line L742 (-10076.322021, -10031.554802) -> (-10079.073422, -10031.693905)
  ellipse E609 centre (-10075.377134, -10011.589397) end of major axis (-10075.590063, -10009.701366) minor radius 0.04047 (-10075.534229, -10010.000611) -> (-10075.57783, -10010.005705) ccw
  ellipse E610 centre (-10078.158864, -10011.903116) end of major axis (-10078.371793, -10010.015085) minor radius 0.04047 (-10078.375381, -10010.064518) -> (-10078.35867, -10010.330575) ccw
  line L743 (-10075.590063, -10009.701366) -> (-10077.531536, -10009.920322)
  ellipse E611 centre (-10075.377134, -10026.604585) end of major axis (-10075.590063, -10028.492616) minor radius 0.04047 (-10075.57783, -10028.188277) -> (-10075.534229, -10028.193371) ccw
  ellipse E612 centre (-10078.158864, -10026.290866) end of major axis (-10078.371793, -10028.178897) minor radius 0.04047 (-10078.35867, -10027.863407) -> (-10078.375381, -10028.129463) ccw
  line L744 (-10075.590063, -10028.492616) -> (-10077.531536, -10028.27366)
  ellipse E613 centre (-10076.417956, -10008.536756) end of major axis (-10076.342218, -10007.038669) minor radius 0.268093 (-10076.196715, -10007.346408) -> (-10076.619894, -10009.817509) ccw
  ellipse E614 centre (-10076.417956, -10008.536756) end of major axis (-10076.322021, -10006.639179) minor radius 0.339584 (-10076.094418, -10007.35158) -> (-10076.730075, -10009.829935) ccw
  ellipse E615 centre (-10079.169358, -10008.397654) end of major axis (-10079.073422, -10006.500077) minor radius 0.339584 (-10079.073422, -10006.500077) -> (-10079.471363, -10007.882293) ccw
  line L745 (-10076.322021, -10006.639179) -> (-10079.073422, -10006.500077)
  ellipse E616 centre (-10080.128023, -10028.828349) end of major axis (-10080.137907, -10027.328382) minor radius 0.235872 (-10080.352426, -10028.304713) -> (-10080.353303, -10028.321891) ccw
  ellipse E617 centre (-10080.128023, -10028.828349) end of major axis (-10080.140543, -10026.92839) minor radius 0.298772 (-10080.418344, -10028.298273) -> (-10080.359687, -10029.968585) ccw
  ellipse E618 centre (-10082.893128, -10028.846569) end of major axis (-10082.880609, -10030.746528) minor radius 0.298772 (-10082.967192, -10030.666579) -> (-10082.880609, -10030.746528) ccw
  line L746 (-10081.422499, -10030.73692) -> (-10082.880609, -10030.746528)
  ellipse E619 centre (-10079.300565, -10011.695557) end of major axis (-10079.485297, -10009.804559) minor radius 0.109208 (-10079.427129, -10009.955048) -> (-10079.514898, -10010.075585) ccw
  ellipse E620 centre (-10082.082692, -10011.967344) end of major axis (-10082.267424, -10010.076346) minor radius 0.109208 (-10082.267424, -10010.076346) -> (-10082.283245, -10010.78891) ccw
  line L747 (-10079.485297, -10009.804559) -> (-10082.267424, -10010.076346)
  ellipse E621 centre (-10079.300565, -10026.498425) end of major axis (-10079.485297, -10028.389423) minor radius 0.109208 (-10079.514898, -10028.118396) -> (-10079.427129, -10028.238934) ccw
  ellipse E622 centre (-10082.082692, -10026.226637) end of major axis (-10082.267424, -10028.117635) minor radius 0.109208 (-10082.283245, -10027.405071) -> (-10082.267424, -10028.117635) ccw
  line L748 (-10079.485297, -10028.389423) -> (-10082.267424, -10028.117635)
  ellipse E623 centre (-10080.128023, -10009.365633) end of major axis (-10080.118139, -10007.865665) minor radius 0.235872 (-10080.353303, -10009.872091) -> (-10080.352426, -10009.889269) ccw
  ellipse E624 centre (-10080.128023, -10009.365633) end of major axis (-10080.115503, -10007.465674) minor radius 0.298772 (-10080.359687, -10008.225397) -> (-10080.418344, -10009.895709) ccw
  ellipse E625 centre (-10082.893128, -10009.347412) end of major axis (-10082.880609, -10007.447453) minor radius 0.298772 (-10082.880609, -10007.447453) -> (-10082.967192, -10007.527403) ccw
  line L749 (-10081.422499, -10007.457061) -> (-10082.880609, -10007.447453)
  line L750 (-10073.916152, -10027.841726) -> (-10073.815719, -10027.825263)
  line L751 (-10073.715814, -10027.808888) -> (-10066.427775, -10026.614286)
  line L752 (-10066.011544, -10022.636001) -> (-10068.219035, -10021.777356)
  line L753 (-10066.011516, -10022.636084) -> (-10066.011544, -10022.636001)
  line L754 (-10079.441685, -10027.263612) -> (-10075.810846, -10027.643492)
  line L755 (-10073.920953, -10027.841223) -> (-10073.916152, -10027.841726)
  line L756 (-10079.441658, -10027.263695) -> (-10078.716426, -10027.339573)
  line L757 (-10066.019037, -10022.707967) -> (-10066.011516, -10022.636084)
  line L758 (-10066.427775, -10026.614286) -> (-10066.383563, -10026.191708)
  line L759 (-10066.210046, -10024.533256) -> (-10066.011544, -10022.636001)
  ellipse E626 centre (-10079.44163, -10027.263778) end of major axis (-10078.936388, -10027.316639) minor radius 0.000079 (-10079.441658, -10027.263695) -> (-10079.67495, -10027.239296) ccw
  ellipse E627 centre (-10079.44163, -10027.263778) end of major axis (-10078.431146, -10027.369501) minor radius 0.000159 (-10079.441686, -10027.263612) -> (-10079.908269, -10027.214814) ccw
  ellipse E628 centre (-10085.955114, -10026.582835) end of major axis (-10086.965599, -10026.477113) minor radius 0.000159 (-10086.421753, -10026.533871) -> (-10086.965599, -10026.477113) ccw
  ellipse E629 centre (-10085.955114, -10026.582835) end of major axis (-10086.460356, -10026.529974) minor radius 0.000079 (-10086.188433, -10026.558353) -> (-10086.460356, -10026.529974) ccw
  line L760 (-10086.965599, -10026.477113) -> (-10086.933123, -10026.166713)
  line L761 (-10079.674949, -10027.239296) -> (-10086.188433, -10026.558353)
  line L762 (-10079.908269, -10027.214814) -> (-10086.421753, -10026.533871)
  line L763 (-10086.965544, -10026.477275) -> (-10087.069431, -10027.472361)
  line L764 (-10086.564188, -10027.525223) -> (-10087.069431, -10027.472361)
  line L765 (-10086.564188, -10027.525223) -> (-10086.460302, -10026.530137)
  line L766 (-10086.965544, -10026.477275) -> (-10086.460302, -10026.530137)
  line L767 (-10087.069431, -10027.472361) -> (-10087.069401, -10027.47245)
  line L768 (-10086.460302, -10026.530137) -> (-10086.460356, -10026.529974)
  line L769 (-10086.965599, -10026.477113) -> (-10086.965544, -10026.477275)
  line L770 (-10080.370226, -10023.096991) -> (-10079.694033, -10023.096991)
  line L771 (-10080.370226, -10015.096991) -> (-10079.694033, -10015.096991)
  line L772 (-10080.370226, -10023.096991) -> (-10080.824868, -10023.096991)
  line L773 (-10080.370226, -10015.096991) -> (-10080.824868, -10015.096991)
  line L774 (-10080.824868, -10023.096991) -> (-10081.297088, -10023.096991)
  line L775 (-10081.297088, -10015.096991) -> (-10080.824868, -10015.096991)
  line L776 (-10087.224014, -10014.775485) -> (-10087.329747, -10015.096991)
  line L777 (-10086.824506, -10015.096991) -> (-10086.739212, -10014.837634)
  line L778 (-10087.329747, -10023.096991) -> (-10087.224014, -10023.418496)
  line L779 (-10086.739212, -10023.356347) -> (-10086.824506, -10023.096991)
  line L780 (-10066.011544, -10015.55798) -> (-10066.011516, -10015.557898)
  line L781 (-10068.219035, -10016.416626) -> (-10066.011544, -10015.55798)
  line L782 (-10066.427775, -10011.579695) -> (-10073.715814, -10010.385094)
  line L783 (-10073.815719, -10010.368718) -> (-10073.916152, -10010.352256)
  line L784 (-10078.716426, -10010.854409) -> (-10079.441658, -10010.930287)
  line L785 (-10079.441685, -10010.930369) -> (-10075.810846, -10010.55049)
  line L786 (-10073.920953, -10010.352758) -> (-10073.916152, -10010.352256)
  line L787 (-10066.011516, -10015.557898) -> (-10066.019037, -10015.486015)
  line L788 (-10066.011544, -10015.55798) -> (-10066.210046, -10013.660726)
  line L789 (-10066.383563, -10012.002274) -> (-10066.427775, -10011.579695)
  ellipse E630 centre (-10079.44163, -10010.930204) end of major axis (-10079.946872, -10010.983065) minor radius 0.000079 (-10079.674949, -10010.954686) -> (-10079.441658, -10010.930287) ccw
  ellipse E631 centre (-10079.44163, -10010.930204) end of major axis (-10078.431146, -10010.824481) minor radius 0.000159 (-10079.908269, -10010.979168) -> (-10079.441686, -10010.930369) ccw
  ellipse E632 centre (-10085.955114, -10011.611146) end of major axis (-10086.965599, -10011.716869) minor radius 0.000159 (-10086.965599, -10011.716869) -> (-10086.421753, -10011.66011) ccw
  ellipse E633 centre (-10085.955114, -10011.611146) end of major axis (-10086.460356, -10011.664008) minor radius 0.000079 (-10086.460356, -10011.664008) -> (-10086.188433, -10011.635628) ccw
  line L790 (-10086.933123, -10012.027269) -> (-10086.965599, -10011.716869)
  line L791 (-10079.674949, -10010.954686) -> (-10086.188433, -10011.635628)
  line L792 (-10086.421753, -10011.66011) -> (-10079.908269, -10010.979168)
  line L793 (-10087.069431, -10010.72162) -> (-10086.965544, -10011.716706)
  line L794 (-10086.460302, -10011.663845) -> (-10086.965544, -10011.716706)
  line L795 (-10086.460302, -10011.663845) -> (-10086.564188, -10010.668759)
  line L796 (-10086.564188, -10010.668759) -> (-10087.069431, -10010.72162)
  line L797 (-10087.069401, -10010.721532) -> (-10087.069431, -10010.72162)